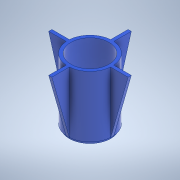
# Autodesk Inventor part: tail
Saved by Autodesk Inventor 2020 (Build 240168000, 168)
## iProperties
Created: 2021-01-23
Part Number: tail
Material: ABS Plastic
Document SubType Name: Modeling
Designer: 0x6f736f646f
Density: 1.06 g/cm^3
Appearance: Smooth - White
Author: 0x6f736f646f
Autodesk Inventor part; units mm, degrees
ref_plane "YZ Plane" through (0, 0, 0) normal (1, 0, 0) x (0, 1, 0)
ref_plane "XZ Plane" through (0, 0, 0) normal (0, 1, 0) x (-1, 0, 0)
ref_plane "XY Plane" through (0, 0, 0) normal (0, 0, 1) x (1, 0, 0)
sketch "Sketch1" plane through (0, 0, 0) normal (0, 1, 0) x (-1, 0, 0)
  circle A0 centre (0, 0) radius 30
  circle A1 centre (0, 0) radius 32.5
  circle A2 centre (0, 0) radius 35
  dimension "d0" = 60
  dimension "d1" = 65
  dimension "d2" = 70
  constraints: 3 centre point, 3 coincident
  measures "d0" diameter of A0
  measures "d1" diameter of A1
  measures "d2" diameter of A2
extrude "Extrusion1" add sketch "Sketch1" along normal blind 96 and the other way blind 4 contours A1
extrude "Extrusion2" add sketch "Sketch1" along normal blind 96 contours A2
sketch "Sketch3" plane through (0, 0, 0) normal (0, 0, 1) x (1, 0, 0)
  line L0 (-32.5, 0) -> (32.5, 0) projected
  line L1 (-32.5, 0) -> (-32.5, 96)
  line L2 (35, 96) -> (-35, 96) projected
  line L3 (-32.5, 96) -> (-62.5, 96)
  line L4 (-62.5, 96) -> (-35, 0)
  line L5 (-35, 0) -> (-35, 96) projected
  line L6 (35, 0) -> (-35, 0) projected
  line L7 (-35, 0) -> (-32.5, 0)
  point P0 (0, 0)
  dimension "d10" = 30
  constraints: 8 end point, 2 point on line, 1 collinear, 1 horizontal, 1 vertical
  measures "d10" distance of L1.end L3.end
extrude "Extrusion3" add sketch "Sketch3" along normal mid plane 5
pattern_circular "Circular Pattern1" count 4 over 360 about axis through (0, -10, 0) along (0, 1, 0) of "Extrusion3"
body "Solid1"
